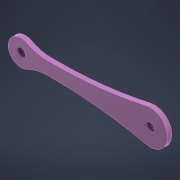
# Autodesk Inventor part: Рычаг_1
Saved by Autodesk Inventor 2021.2 (Build 252289000, 289)
## iProperties
Created: 2021-05-30
Part Number: Рычаг_1
Material: Типовые
Document SubType Name: Modeling
Designer: Admin
Density: 1 g/cm^3
Appearance: Гладкий - пурпурный
Mass: 21.1786 g
Surface Area: 108.568 cm^2
Volume: 21.1786 cm^3
Author: Admin
Autodesk Inventor part; units mm, degrees
ref_plane "YZ Plane" through (0, 0, 0) normal (1, 0, 0) x (0, 1, 0)
ref_plane "XZ Plane" through (0, 0, 0) normal (0, 1, 0) x (-1, 0, 0)
ref_plane "XY Plane" through (0, 0, 0) normal (0, 0, 1) x (1, 0, 0)
sketch "Эскиз1" plane through (0, 0, 0) normal (0, 0, 1) x (1, 0, 0)
  arc A0 (6.9948, 13.2692) -> (6.9948, -13.2692) centre (0, 0) ccw
  line L0 (30.3109, 7.5) -> (36.6697, 7.5)
  line L1 (30.3109, -7.5) -> (36.6697, -7.5)
  arc A1 (145.6411, -19.5192) -> (145.6411, 19.5192) centre (150, 0) ccw
  arc A2 (6.9948, 13.2692) -> (30.3109, 7.5) centre (30.3109, 57.5) ccw
  arc A3 (30.3109, -7.5) -> (6.9948, -13.2692) centre (30.3109, -57.5) ccw
  arc A4 (36.6697, 7.5) -> (145.6411, 19.5192) centre (36.6697, 507.5) ccw
  arc A5 (145.6411, -19.5192) -> (36.6697, -7.5) centre (36.6697, -507.5) ccw
  point P0 (12.9904, 7.5)
  point P1 (131.4595, 7.5)
  point P2 (12.9904, -7.5)
  point P3 (131.4595, -7.5)
  point P4 (-12.9904, 7.5)
  point P5 (-12.9904, -7.5)
  point P6 (131.4595, -7.5)
  point P7 (131.4595, 7.5)
  point P8 (12.9904, 7.5)
  point P9 (12.9904, -7.5)
  dimension "d0" = 30
  dimension "d1" = 40
  dimension "d5" = 150
  dimension "d17" = 15
  dimension "d19" = 50
  dimension "d20" = 500
  constraints: 22 point on circle, 8 point on line, 8 tangent, 6 centre point, 4 end point, 2 equal radius, 2 vertical alignment, 1 coincident, 1 horizontal alignment
  measures "d0" diameter of A0
  measures "d1" diameter of A1
  measures "d5" distance of point (0, 0) A1.centre
  measures "d17" distance between parallel lines of L1 L0
  measures "d19" radius of A2
  measures "d20" radius of A4
extrude "Выдавливание1" add sketch "Эскиз1" along normal blind 5
sketch "Эскиз2" plane through (0, 0, 5) normal (0, 0, 1) x (1, 0, 0)
  arc A0 (145.6411, -19.5192) -> (145.6411, 19.5192) centre (150, 0) ccw projected
  point P0 (0, 0)
  point P1 (0, 0)
  point P2 (88.8197, -10)
  point P3 (88.8197, 10)
  point P4 (142.2738, -12.8571)
  point P5 (142.2738, 12.8571)
  constraints: 2 coincident
hole "Отверстие1" at (0, 0, 5) at (150, 0, 5) direction (0, 0, -1) diameter 10 end through all
